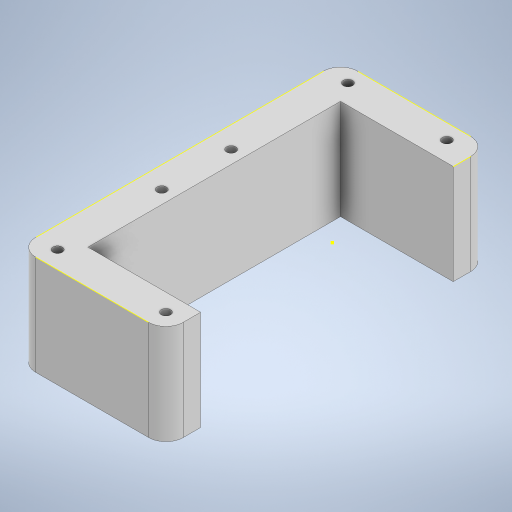
# Autodesk Inventor part: SwerveBH
Saved by Autodesk Inventor 2024 (Build 280153000, 153)
## iProperties
Created: 2023-08-02
Part Number: SwerveBH
Material: Generic
Document SubType Name: Modeling
Designer: s137416
Density: 1 g/cm^3
Appearance: Default
Author: s137416
Title: BH#3
Autodesk Inventor part; units mm, degrees
ref_plane "YZ Plane" through (0, 0, 0) normal (1, 0, 0) x (0, 1, 0)
ref_plane "XZ Plane" through (0, 0, 0) normal (0, 1, 0) x (-1, 0, 0)
ref_plane "XY Plane" through (0, 0, 0) normal (0, 0, 1) x (1, 0, 0)
sketch "Sketch1" plane through (0, 0, 0) normal (0, 1, 0) x (-1, 0, 0)
  line L0 (-82.55, 88.9) -> (82.55, 88.9)
  line L1 (82.55, 88.9) -> (82.55, -88.9)
  line L2 (82.55, -88.9) -> (-82.55, -88.9)
  line L3 (-82.55, -88.9) -> (-82.55, 88.9)
  line L4 (-82.55, 88.9) -> (82.55, -88.9) construction
  line L5 (82.55, 88.9) -> (-82.55, -88.9) construction
  line L6 (4.079, 92.4026) -> (105.679, 92.4026)
  line L7 (105.679, 92.4026) -> (105.679, 117.8026)
  line L8 (105.679, 117.8026) -> (4.079, 117.8026)
  line L9 (4.079, 117.8026) -> (4.079, 92.4026)
  line L10 (111.9367, -9.1974) -> (86.5367, -9.1974)
  line L11 (86.5367, -9.1974) -> (86.5367, 117.8026)
  line L12 (86.5367, 117.8026) -> (111.9367, 117.8026)
  line L13 (111.9367, 117.8026) -> (111.9367, -9.1974)
  line L14 (4.079, -92.4026) -> (105.679, -92.4026)
  line L15 (105.679, -92.4026) -> (105.679, -117.8026)
  line L16 (105.679, -117.8026) -> (4.079, -117.8026)
  line L17 (4.079, -117.8026) -> (4.079, -92.4026)
  line L18 (86.5367, -117.8026) -> (111.9367, -117.8026)
  line L19 (111.9367, -117.8026) -> (111.9367, 9.1974)
  line L20 (111.9367, 9.1974) -> (86.5367, 9.1974)
  line L21 (86.5367, 9.1974) -> (86.5367, -117.8026)
  point P0 (0, 0)
  point P1 (105.679, -117.8026)
  point P2 (86.5367, -92.4026)
  point P3 (86.5367, 92.4026)
  dimension "d0" = 165.1
  dimension "d1" = 177.8
  dimension "d2" = 101.6
  dimension "d3" = 25.4
  dimension "d4" = 25.4
  dimension "d5" = 19.1423
  dimension "d6" = 3.5026
  dimension "d7" = 3.5026
  dimension "d8" = 101.6
  dimension "d9" = 25.4
  dimension "d10" = 25.4
  dimension "d12" = 127
  dimension "d13" = 127
  constraints: 44 end point, 9 parallel, 5 horizontal, 5 perpendicular, 2 midpoint, 2 point on line, 1 collinear
  measures "d0" distance of L1.end L2.end
  measures "d1" distance of L0.end L1.end
  measures "d2" distance of L8.end L7.end
  measures "d3" distance of L6.end L7.end
  measures "d4" distance of L10.start L10.end
  measures "d5" distance between parallel lines of L11 L7
  measures "d6" distance between parallel lines of L6 L0
  measures "d7" distance between parallel lines of L2 L14
  measures "d8" distance of L15.end L16.end
  measures "d9" distance of L14.end L15.end
  measures "d10" distance of L20.end L19.end
  measures "d12" distance of L12.end L10.start
  measures "d13" distance of L18.end L19.end
extrude "Extrusion1" add sketch "Sketch1" along normal blind 73.025 contours L9 L8 L11 L6 | L11 L8 L7 L6 | L6 L7 L12 L13 L20 L11 | L20 L13 L10 L11 | L10 L19 L18 L15 L14 L21 | L21 L16 L17 L14 | L14 L15 L16 L21
fillet "Fillet1" radius 12.7 1 edges at (-111.9367, 36.5125, 117.8026)
fillet "Fillet2" radius 12.7 3 edges at (-111.9367, 36.5125, -117.8026) (-4.079, 36.5125, 117.8026) (-4.079, 36.5125, -117.8026)
sketch "Sketch4" plane through (0, 73.025, 0) normal (0, 1, 0) x (1, 0, 0)
  line L0 (-99.2367, -117.8026) -> (-16.779, -117.8026) projected
  line L1 (-111.9367, 105.1026) -> (-111.9367, -105.1026) projected
  line L2 (-16.779, 117.8026) -> (-99.2367, 117.8026) projected
  line L3 (-4.079, 92.4026) -> (-4.079, 105.1026) projected
  point P0 (0, 0)
sketch "Sketch5" plane through (0, 73.025, 0) normal (0, 1, 0) x (1, 0, 0)
  line L0 (-99.2367, -117.8026) -> (-16.779, -117.8026) projected
  line L1 (-111.9367, 105.1026) -> (-111.9367, -105.1026) projected
  line L2 (-4.079, -105.1026) -> (-4.079, -92.4026) projected
  line L3 (-16.779, 117.8026) -> (-99.2367, 117.8026) projected
  line L4 (-86.5367, 92.4026) -> (-4.079, 92.4026) projected
  circle A0 centre (-96.0617, -105.1026) radius 3.3782
  circle A1 centre (-16.779, -105.1026) radius 3.3782
  circle A2 centre (-96.0617, -28.9026) radius 3.3782
  circle A3 centre (-96.0617, 21.8974) radius 3.3782
  circle A4 centre (-23.0367, 106.6901) radius 3.3782
  circle A5 centre (-95.4047, 106.6901) radius 3.3782
  point P0 (0, 0)
  dimension "d52" = 12.7
  dimension "d53" = 15.875
  dimension "d54" = 12.7
  dimension "d55" = 12.7
  dimension "d56" = 88.9
  dimension "d57" = 139.7
  dimension "d61" = 88.9
  dimension "d62" = 14.2875
  dimension "d63" = 6.7564
  dimension "d64" = 6.7564
  dimension "d65" = 6.7564
  dimension "d66" = 6.7564
  dimension "d67" = 6.7564
  dimension "d73" = 11.1125
  dimension "d74" = 6.7564
  constraints: 6 centre point, 6 coincident
  measures "d52" distance from line of L0 point (-96.062, -105.103)
  measures "d53" distance from line of L1 point (-96.062, -105.103)
  measures "d54" distance from line of L0 point (-16.779, -105.103)
  measures "d55" distance from line of L2 point (-16.779, -105.103)
  measures "d56" distance from line of L0 point (-96.062, -28.903)
  measures "d57" distance from line of L0 point (-96.062, 21.897)
  measures "d61" distance from line of L1 point (-23.037, 106.69)
  measures "d62" distance from line of L4 point (-23.037, 106.69)
  measures "d63" diameter of A0
  measures "d64" diameter of A1
  measures "d65" diameter of A2
  measures "d66" diameter of A3
  measures "d67" diameter of A4
  measures "d73" distance from line of L3 point (-95.405, 106.69)
  measures "d74" diameter of A5
extrude "Extrusion4" cut sketch "Sketch5" against normal through all
body "Solid1"
